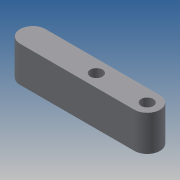
# Autodesk Inventor part: ARM
Saved by Autodesk Inventor 2013 (Build 170138000, 138)
## iProperties
Created: 2017-02-24
Part Number: ARM
Material: Generic
Document SubType Name: Modeling
Designer: employee
Density: 1 g/cm^3
Author: employee
Autodesk Inventor part; units mm, degrees
ref_plane "YZ Plane" through (0, 0, 0) normal (1, 0, 0) x (0, 1, 0)
ref_plane "XZ Plane" through (0, 0, 0) normal (0, 1, 0) x (-1, 0, 0)
ref_plane "XY Plane" through (0, 0, 0) normal (0, 0, 1) x (1, 0, 0)
sketch "Sketch1" plane through (0, 0, 0) normal (0, 0, 1) x (1, 0, 0)
  line L0 (0, 12.5) -> (112.5, 12.5)
  arc A0 (112.5, -12.5) -> (112.5, 12.5) centre (112.5, 0) ccw
  line L1 (112.5, -12.5) -> (0, -12.5)
  arc A1 (0, 12.5) -> (0, -12.5) centre (0, 0) ccw
  dimension "d0" = 25
  dimension "d2" = 112.5
  constraints: 4 end point, 4 point on circle, 4 tangent, 2 centre point, 1 coincident, 1 horizontal, 1 parallel
  measures "d0" distance between parallel lines of L1 L0
  measures "d2" distance of L0.start L0.end
extrude "Extrusion1" add sketch "Sketch1" along normal mid plane 35
sketch "Sketch2" plane through (0, 0, 17.5) normal (0, 0, 1) x (1, 0, 0)
  arc A0 (112.5, -12.5) -> (112.5, 12.5) centre (112.5, 0) ccw projected
  circle A1 centre (112.5, 0) radius 6
  circle A2 centre (62.5, 0) radius 6
  dimension "d5" = 12
  dimension "d7" = 50
  constraints: 2 centre point, 1 coincident, 1 equal radius, 1 horizontal alignment
  measures "d5" diameter of A1
  measures "d7" distance of A0.centre A2.centre
extrude "Extrusion2" cut sketch "Sketch2" against normal through all
body "Solid1"
